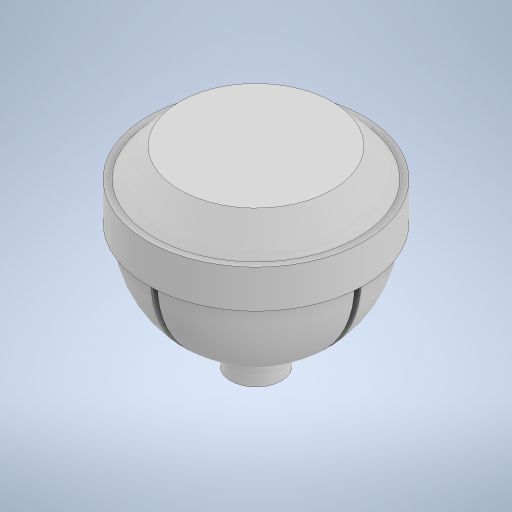
# Autodesk Inventor part: 屋1 物1 base
Saved by Autodesk Inventor 2024 (Build 280153000, 153)
## iProperties
Created: 2024-05-23
Part Number: 屋1 物1 base
Material: 一般
Document SubType Name: Modeling
Designer: User
Density: 1 g/cm^3
Appearance: 預設
Author: User
Autodesk Inventor part; units mm, degrees
ref_plane "YZ Plane" through (0, 0, 0) normal (1, 0, 0) x (0, 1, 0)
ref_plane "XZ Plane" through (0, 0, 0) normal (0, 1, 0) x (-1, 0, 0)
ref_plane "XY Plane" through (0, 0, 0) normal (0, 0, 1) x (1, 0, 0)
sketch "草圖1" plane through (0, 0, 0) normal (0, 0, 1) x (1, 0, 0)
  line L0 (0, 0) -> (12, 0)
  line L1 (12, 0) -> (16, -4.5023)
  line L2 (16, -4.5023) -> (0, -4.5023)
  line L3 (0, 0) -> (0, -4.5023)
  dimension "d0" = 12
  dimension "d1" = 16
  constraints: 8 end point, 1 horizontal, 1 parallel, 1 vertical
  measures "d0" distance of L0.start L0.end
  measures "d1" distance of L2.end L1.end
revolve "迴轉1" add sketch "草圖1" angle 360 about axis through (0, 0, 0) along (0, -1, 0)
sketch "草圖2" plane through (0, -4.5023, 0) normal (0, -1, 0) x (1, 0, 0)
  circle A0 centre (0, 0) radius 17
  dimension "d3" = 34
  constraints: 1 centre point, 1 coincident
  measures "d3" diameter of A0
extrude "擠出1" add sketch "草圖2" along normal blind 6
sketch "草圖3" plane through (0, -10.5023, 0) normal (0, -1, 0) x (1, 0, 0)
  circle A0 centre (0, 0) radius 16
  circle A1 centre (0, 0) radius 16 projected
  line L0 (0, 16) -> (0, -16)
  dimension "d6" = 32
  constraints: 2 end point, 2 point on circle, 1 centre point, 1 coincident
  measures "d6" diameter of A0
revolve "迴轉2" add sketch "草圖3" angle 180 about axis through (0, -10.5023, 16) along (0, 0, -1) picked at (2.314, 4.8052) contours A0 L0
sketch "草圖4" plane through (0, 0, 0) normal (0, 0, 1) x (1, 0, 0)
  arc A0 (-16, -10.5023) -> (16, -10.5023) centre (0, -10.5023) ccw projected
  arc A1 (-16, -10.5023) -> (16, -10.5023) centre (0, -10.5023) ccw
  line L0 (-17, -10.5023) -> (17, -10.5023) projected
  arc A2 (-15, -10.5023) -> (15, -10.5023) centre (0, -10.5023) ccw
  line L1 (-16, -10.5023) -> (-15, -10.5023)
  line L2 (15, -10.5023) -> (16, -10.5023)
  point P0 (0, 0)
  dimension "d8" = 1
  constraints: 6 point on circle, 4 end point, 2 centre point, 2 collinear, 2 point on line, 1 concentric
  measures "d8" radial gap between concentric circles of A0 A2
extrude "擠出2" cut sketch "草圖4" along normal mid plane 1 contours L0 A2 A0
sketch "草圖5" plane through (0, 0, 0) normal (1, 0, 0) x (0, 1, 0)
  arc A0 (-10.5023, 16) -> (-26.4945, 0.5) centre (-10.5023, 0) ccw projected
  arc A1 (-26.4945, -0.5) -> (-10.5023, -16) centre (-10.5023, 0) ccw projected
  arc A2 (-10.5023, 16) -> (-10.5023, -16) centre (-10.5023, 0) ccw
  line L0 (-10.5023, -16) -> (-10.5023, -0.5) projected
  arc A3 (-10.5023, 15) -> (-10.5023, -15) centre (-10.5023, 0) ccw
  line L1 (-10.5023, -16) -> (-10.5023, -15)
  line L2 (-10.5023, 16) -> (-10.5023, 15)
  line L3 (-10.5023, 17) -> (-10.5023, -17) projected
  point P0 (0, 0)
  point P1 (-26.4945, 0.5)
  point P2 (-26.4945, -0.5)
  dimension "d11" = 1
  constraints: 6 point on circle, 4 end point, 2 centre point, 2 collinear, 1 concentric, 1 point on line
  measures "d11" radial gap between concentric circles of A0 A3
extrude "擠出3" cut sketch "草圖5" along normal mid plane 1 contours L2 A3 L0 A1 A2 A0
sketch "草圖6" plane through (0, 0, 0) normal (0, 1, 0) x (1, 0, 0)
  line L0 (0.5, -0.5) -> (0, 0) projected
  circle A0 centre (0, 0) radius 4
  dimension "d14" = 8
  constraints: 1 centre point, 1 coincident
  measures "d14" diameter of A0
extrude "擠出4" add sketch "草圖6" against normal blind 30
